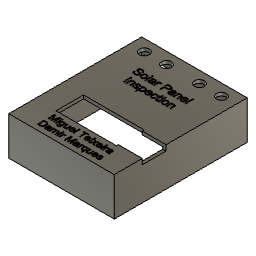
Earpiece v3 (Autodesk Fusion 360 design; units mm, degrees)
Autodesk Fusion 360 part; units mm, degrees
sketch "Esboço1" plane through (0, 0, 0) normal (0, 0, 1) x (1, 0, 0)
  line L0 (45, 57.5) -> (-45, 57.5)
  line L1 (-45, 57.5) -> (-45, -57.5)
  line L2 (-45, -57.5) -> (45, -57.5)
  line L3 (45, -57.5) -> (45, 57.5)
  line L4 (45, 57.5) -> (-45, -57.5) construction
  line L5 (-45, 57.5) -> (45, -57.5) construction
  circle A0 centre (-35, 50) radius 4.5
  circle A1 centre (35, 50) radius 4.5
  circle A2 centre (-15, 50) radius 4.5
  circle A3 centre (15, 50) radius 4.5
  line L6 (26.2799, -11.6979) -> (-28.7201, -11.6979)
  line L7 (-28.7201, -11.6979) -> (-28.7201, -36.6979)
  line L8 (-28.7201, -36.6979) -> (26.2799, -36.6979)
  line L9 (26.2799, -36.6979) -> (26.2799, -11.6979)
  line L10 (48, -60.5) -> (-48, -60.5)
  line L11 (-48, -60.5) -> (-48, 60.5)
  line L12 (-48, 60.5) -> (48, 60.5)
  line L13 (48, 60.5) -> (48, -60.5)
  line L14 (48, -60.5) -> (-48, 60.5) construction
  line L15 (-48, -60.5) -> (48, 60.5) construction
  line L16 (-35, 5) -> (35, 5) construction
  line L17 (35, 5) -> (35, 35) construction
  line L18 (35, 35) -> (-35, 35) construction
  line L19 (-35, 35) -> (-35, 5) construction
  line L20 (-40.1342, -54.8573) -> (42.9318, -54.8573) construction
  line L21 (42.9318, -54.8573) -> (42.9318, -40.2628) construction
  line L22 (42.9318, -40.2628) -> (-40.1342, -40.2628) construction
  line L23 (-40.1342, -40.2628) -> (-40.1342, -54.8573) construction
  line L24 (25, -13.3979) -> (48, -13.3979)
  line L25 (48, -34.9979) -> (25, -34.9979)
  line L26 (25, -34.9979) -> (25, -13.3979)
  dimension "d9" = 90
  dimension "d10" = 115
  dimension "d11" = 9
  dimension "d12" = 9
  dimension "d13" = 9
  dimension "d14" = 9
  dimension "d16" = 55
  dimension "d17" = 25
  dimension "d33" = 7
  dimension "d37" = 6
  dimension "d41" = 3
  dimension "d42" = 3
  dimension "d43" = 1.7
  dimension "d44" = 1.7
  text T0 "Solar Panel Inspection" font "Arial" height 7 align centre top in box 70 x 30 at (-35, 5) x (1, 0) y (0, 1) spacing 1
  text T1 "Miguel Teixeira\nDamir Marques" font "Arial" height 6 align centre top in box 83.066 x 14.5946 at (-40.1342, -54.8573) x (1, 0) y (0, 1) spacing 1
  constraint horizontal L0
  constraint perpendicular L0 L1
  constraint parallel L0 L2
  constraint parallel L1 L3
  constraint coincident L4 origin
  constraint coincident L5 origin
  constraint horizontal L6
  constraint vertical L7
  constraint horizontal L8
  constraint vertical L9
  constraint coincident L4 L7.end
  constraint horizontal L10
  constraint perpendicular L10 L11
  constraint parallel L10 L12
  constraint parallel L11 L13
  constraint coincident L14 origin
  constraint coincident L15 origin
  constraint coincident L5
  constraint horizontal L24
  constraint horizontal L25
  constraint vertical L26
  constraint coincident L13 L25.start
  measures "d9" distance of L1.end L2.end
  measures "d10" distance of L0.start L2.end
  measures "d11" diameter of A0
  measures "d12" diameter of A1
  measures "d13" diameter of A2
  measures "d14" diameter of A3
  measures "d16" distance of L6.start L6.end
  measures "d17" distance of L6.start L8.end
  measures "d41" distance of L1 L11
  measures "d42" distance of L0 L12
  measures "d43" distance of L6 L24
  measures "d44" distance of L8 L25
extrude "Extrusão6" add sketch "Esboço1" along normal blind 35 contours L0 L1 L2 L3 L6 L7 L8 L9 L24 L25 | L0 L1 L2 L3 L10 L11 L12 L13 L24 L25 | L3 L13 L24 L25 | L3 L9 L24 L25 | L6 L7 L8 L9 L24 L25 L26 | L9 L24 L25 L26 | A0 | A1 | A2 | A3
extrude "Extrusão7" cut sketch "Esboço1" along normal blind 32 contours L0 L1 L2 L3 L6 L7 L8 L9 L24 L25 | L3 L9 L24 L25 | L6 L7 L8 L9 L24 L25 L26 | L9 L24 L25 L26 | A0 | A1 | A2 | A3
extrude "Extrusão8" cut sketch "Esboço1" against normal blind 35 from surface at 35 contours L6 L7 L8 L9 L24 L25 L26 | L9 L24 L25 L26
extrude "Extrusão9" cut sketch "Esboço1" against normal blind 30 from surface at 35 contours A0 | A1 | A2 | A3
extrude "Extrusão10" cut sketch "Esboço1" against normal blind 1 from surface at 35 text T0
extrude "Extrusão11" cut sketch "Esboço1" against normal blind 1 from surface at 35 text T1
extrude "Extrusão12" cut sketch "Esboço1" against normal blind 5 from surface at 35 contours L3 L9 L24 L25 | L9 L24 L25 L26
extrude "Extrusão13" cut sketch "Esboço1" against normal blind 5 from surface at 35 contours L3 L13 L24 L25 | L3 L9 L24 L25
sketch "Esboço3" plane through (0, 60.5, 0) normal (0, 1, 0) x (-1, 0, 0)
  line L0 (-48, 0) -> (48, 0)
  line L1 (48, 0) -> (48, 35)
  line L2 (48, 35) -> (-48, 35)
  line L3 (-48, 35) -> (-48, 0)
  line L4 (43, 0) -> (13, 0)
  line L5 (13, 0) -> (13, 25)
  line L6 (13, 25) -> (43, 25)
  line L7 (43, 25) -> (43, 0)
  dimension "d51" = 30
  dimension "d52" = 25
  constraint horizontal L4
  constraint vertical L5
  constraint horizontal L6
  constraint vertical L7
  constraint coincident L0 L4.start
  measures "d51" distance of L5.end L6.end
  measures "d52" distance of L4.start L6.end
extrude "Extrusão14" cut sketch "Esboço3" against normal blind 115 contours L0 L4 L5 L6 L7
equation "d42 = d41"
